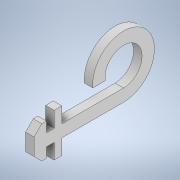
# Autodesk Inventor part: cable holder
Saved by Autodesk Inventor 2020 (Build 240168000, 168)
## iProperties
Created: 2020-01-06
Part Number: cable holder
Material: Générique
Document SubType Name: Modeling
Designer: damien
Density: 1 g/cm^3
Appearance: Par défaut
Author: damien
Autodesk Inventor part; units mm, degrees
ref_plane "YZ Plane" through (0, 0, 0) normal (1, 0, 0) x (0, 1, 0)
ref_plane "XZ Plane" through (0, 0, 0) normal (0, 1, 0) x (-1, 0, 0)
ref_plane "XY Plane" through (0, 0, 0) normal (0, 0, 1) x (1, 0, 0)
sketch "Esquisse1" plane through (0, 0, 0) normal (1, 0, 0) x (0, 1, 0)
  line L0 (-5.5, 0) -> (5.5, 0)
  line L1 (10.5, -8) -> (4, -8)
  line L2 (4, -8) -> (4, -13)
  line L3 (4, -13) -> (14, -13)
  line L4 (14, -13) -> (14, -18)
  line L5 (14, -18) -> (4, -18)
  arc A0 (4, -58) -> (14, -46.1678) centre (16, -58) ccw
  arc A1 (-4, -58) -> (14, -38.1003) centre (16, -58) ccw
  line L6 (-10.5, -8) -> (-4, -8)
  line L7 (-4, -8) -> (-4, -13)
  line L8 (-4, -13) -> (-14, -13)
  line L9 (-14, -13) -> (-14, -18)
  line L10 (-14, -18) -> (-4, -18)
  line L11 (4, -18) -> (4, -58)
  line L12 (-4, -18) -> (-4, -58)
  line L13 (5.5, 0) -> (10.5, -5)
  line L14 (10.5, -5) -> (10.5, -8)
  line L15 (-5.5, 0) -> (-10.5, -5)
  line L16 (-10.5, -5) -> (-10.5, -8)
  line L17 (14, -38.1003) -> (14, -46.1678)
  point P0 (0, 0)
  point P1 (0, 0)
  dimension "d0" = 8
  dimension "d1" = 8
  dimension "d2" = 3
  dimension "d3" = 10
  dimension "d4" = 8
  dimension "d5" = 40
  dimension "d6" = 5
  dimension "d7" = 5
  dimension "d8" = 40
  dimension "d9" = 10
  dimension "d10" = 21
  dimension "d11" = 45
  constraints: 37 end point, 8 perpendicular, 6 equal length, 4 point on circle, 4 vertical, 2 centre point, 2 coincident, 2 horizontal, 2 parallel, 2 point on line, 1 collinear, 1 midpoint, 1 tangent
  measures "d0" distance between parallel lines of L7 L2
  measures "d1" distance between parallel lines of L1 L0
  measures "d2" distance of L13.end L1.start
  measures "d3" distance of L4.end L5.end
  measures "d4" radial gap between concentric circles of A0 A1
  measures "d5" diameter of A1
  measures "d6" distance between parallel lines of L5 L3
  measures "d7" distance of L1.end L2.end
  measures "d8" distance from line of A0.centre L5
  measures "d9" distance between parallel lines of L11 L17
  measures "d10" distance between parallel lines of L16 L14
  measures "d11" angle of L16 L15
extrude "Extrusion1" add sketch "Esquisse1" along normal blind 5.5
